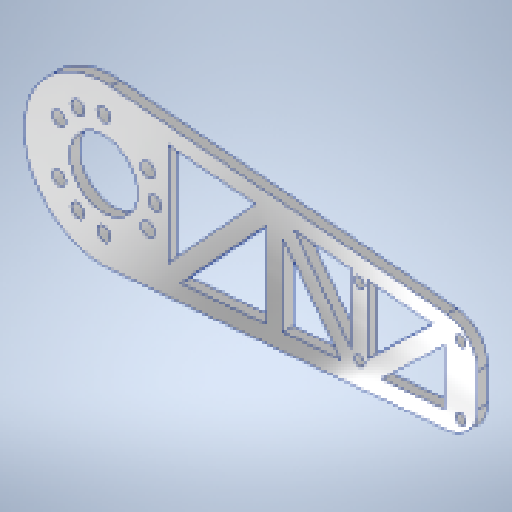
# Autodesk Inventor part: link1plate4
Saved by Autodesk Inventor 2024 (Build 280153000, 153)
## iProperties
Created: 2025-02-07
Part Number: link1plate4
Material: アルミニウム 6061
Document SubType Name: Modeling
Designer: tanoue_kota
Mass: 24.6432 g
Surface Area: 89.3933 cm^2
Volume: 9.1271 cm^3
Density: 2.7 g/cm^3
Appearance: アルミニウム - フラット
Author: tanoue_kota
Autodesk Inventor part; units mm, degrees
ref_plane "YZ Plane" through (0, 0, 0) normal (1, 0, 0) x (0, 1, 0)
ref_plane "XZ Plane" through (0, 0, 0) normal (0, 1, 0) x (-1, 0, 0)
ref_plane "XY Plane" through (0, 0, 0) normal (0, 0, 1) x (1, 0, 0)
sketch "スケッチ1" plane through (0, 0, 0) normal (0, 0, 1) x (1, 0, 0)
  line L0 (0, 0) -> (-57.5, 0)
  line L1 (-57.5, 0) -> (-57.5, 28)
  line L2 (-57.5, 28) -> (0, 28)
  line L3 (0, 28) -> (0, 0)
  line L4 (0, 14) -> (-110.5, 14)
  circle A0 centre (-110.5, 14) radius 53
  circle A1 centre (-110.5, 14) radius 23.5
  line L5 (0, 28) -> (-108.4685, 37.412)
  line L6 (0, 0) -> (-108.4685, -9.412)
  point P0 (-108.4685, -9.412)
  dimension "d3" = 47
  dimension "d0" = 28
  dimension "d1" = 57.5
  dimension "d2" = 106
  constraints: 14 end point, 2 coincident, 2 horizontal, 2 parallel, 1 centre point, 1 midpoint, 1 perpendicular, 1 symmetric about line, 1 tangent, 4 other
  measures "d0" distance of L2.end L0.start
  measures "d1" distance of L1.end L2.end
  measures "d2" diameter of A0
extrude "押し出し1" add sketch "スケッチ1" along normal blind 3 contours L6 A0 L1 L0 | L0 L1 L4 L3 | L4 L1 L2 L3 | L6 A1 L4 A0 | A0 L5 L2 L1 | L4 A1 L5 A0 | A1
sketch "スケッチ2" plane through (0, 0, 3) normal (0, 0, 1) x (1, 0, 0)
  line L0 (0, 28) -> (-108.4685, 37.412) projected
  line L1 (0, 28) -> (-47.5, 28)
  line L2 (-47.5, 28) -> (-47.5, 0)
  line L3 (-47.5, 0) -> (0, 0)
  line L4 (0, 0) -> (0, 28)
  line L5 (-5, 28) -> (-5, 0)
  line L6 (-35, 28) -> (-35, 0)
  line L7 (0, 14) -> (-47.5, 14)
  point P0 (-35, 24)
  point P1 (-5, 24)
  point P2 (-35, 4)
  point P3 (-5, 4)
  dimension "d6" = 28
  dimension "d7" = 47.5
  dimension "d8" = 5
  dimension "d9" = 30
  dimension "d10" = 10
  dimension "d11" = 10
  constraints: 14 end point, 6 point on line, 3 perpendicular, 2 midpoint, 2 parallel, 2 symmetric about line, 1 horizontal
  measures "d6" distance between parallel lines of L1 L3
  measures "d7" distance between parallel lines of L4 L2
  measures "d8" distance between parallel lines of L4 L5
  measures "d9" distance between parallel lines of L5 L6
  measures "d10" distance from line of L7 point (-5, 24)
  measures "d11" distance from line of L7 point (-35, 24)
hole "穴1" at (-35, 24, 3) at (-5, 24, 3) at (-35, 4, 3) at (-5, 4, 3) direction (0, 0, -1) diameter 3.1 end through all
sketch "スケッチ3" plane through (0, 0, 3) normal (0, 0, 1) x (1, 0, 0)
  arc A0 (-108.4685, 37.412) -> (-108.4685, -9.412) centre (-110.5, 14) ccw projected
  circle A1 centre (-110.5, 14) radius 15.18
  circle A2 centre (-110.5, 14) radius 6
  line L0 (-110.5, 14) -> (-118.09, 27.1463)
  line L1 (-123.6463, 21.59) -> (-110.5, 14)
  line L2 (-110.5, 14) -> (-102.91, 27.1463)
  line L3 (-110.5, 14) -> (-110.5, 29.18)
  point P0 (0, 0)
  point P1 (-123.6463, 6.41)
  point P2 (-110.5, -1.18)
  point P3 (-97.3537, 6.41)
  point P4 (-97.3537, 21.59)
  point P5 (-110.5, 29.18)
  point P6 (-118.09, 0.8537)
  point P7 (-95.32, 14)
  dimension "d19" = 30.36
  dimension "d22" = 360
  dimension "d24" = 12
  dimension "d28" = 360
  dimension "d59" = 30
  dimension "d61" = 30
  constraints: 8 end point, 4 coincident, 4 point on circle, 2 centre point, 1 perpendicular, 1 vertical, 11 other
  measures "d19" diameter of A1
  measures "d24" diameter of A2
  measures "d59" angle of L0 L1
  measures "d61" angle of L3 L2
hole "穴2" at (-123.6463, 21.59, 3) at (-123.6463, 6.41, 3) at (-110.5, -1.18, 3) at (-97.3537, 6.41, 3) at (-97.3537, 21.59, 3) at (-110.5, 29.18, 3) at (-118.09, 27.1463, 3) at (-118.09, 0.8537, 3) at (-95.32, 14, 3) direction (0, 0, -1) diameter 4.1 end through all
sketch "スケッチ4" plane through (0, 0, 3) normal (0, 0, 1) x (1, 0, 0)
  arc A0 (-108.4685, 37.412) -> (-108.4685, -9.412) centre (-110.5, 14) ccw projected
  circle A1 centre (-110.5, 14) radius 10
  circle A2 centre (-110.5, 14) radius 23.5
  line L0 (-94.4636, -3.178) -> (0, 5.0188)
  line L1 (0, 0) -> (0, 28) projected
  line L2 (-108.4685, -9.412) -> (0, 0) projected
  line L3 (-94.4636, 31.178) -> (0, 22.9812)
  line L4 (0, 28) -> (-108.4685, 37.412) projected
  line L5 (-10, 23.8489) -> (-10, 4.1511)
  line L6 (-37.5, 26.2352) -> (-37.5, 1.7648)
  circle A3 centre (-35, 4) radius 1.55 projected
  line L7 (-32.5, 25.8013) -> (-32.5, 2.1987)
  circle A4 centre (-35, 24) radius 1.55 projected
  line L8 (-10, 23.8489) -> (-32.5, 2.1987)
  line L9 (-32.5, 5.6681) -> (-13.3073, 24.1359)
  line L10 (-28.537, 2.5426) -> (-10, 20.3795)
  line L11 (-62.5, 28.4045) -> (-62.5, -0.4045)
  line L12 (-57.5, 27.9706) -> (-57.5, 0.0294)
  line L13 (-57.5, 27.9706) -> (-37.5, 1.7648)
  line L14 (-57.5, 23.8499) -> (-40.4496, 1.5089)
  line L15 (-54.1321, 27.6784) -> (-37.5, 5.8856)
  line L16 (-94.4636, 31.178) -> (-94.4636, -3.178)
  line L17 (-91.4636, 30.9177) -> (-91.4636, -2.9177)
  line L18 (-62.5, 28.4045) -> (-91.4636, -2.9177)
  line L19 (-91.4636, 0.7646) -> (-65.6521, 28.678)
  line L20 (-87.7615, -2.5965) -> (-62.5, 24.7222)
  dimension "d37" = 20
  dimension "d38" = 5
  dimension "d39" = 5
  dimension "d40" = 10
  dimension "d41" = 2.5
  dimension "d42" = 2.5
  dimension "d43" = 2.5
  dimension "d44" = 2.5
  dimension "d45" = 5
  dimension "d46" = 20
  dimension "d47" = 2.5
  dimension "d48" = 2.5
  dimension "d49" = 3
  dimension "d50" = 2.5
  dimension "d51" = 2.5
  constraints: 32 end point, 8 parallel, 8 point on line, 4 vertical, 3 point on circle, 2 centre point, 2 coincident, 26 other
  measures "d37" diameter of A1
  measures "d40" distance between parallel lines of L1 L5
  measures "d41" distance from line of A3.centre L6
  measures "d42" distance from line of A4.centre L7
  measures "d43" distance between parallel lines of L8 L9
  measures "d44" distance between parallel lines of L8 L10
  measures "d45" distance between parallel lines of L11 L12
  measures "d46" distance between parallel lines of L6 L12
  measures "d47" distance between parallel lines of L13 L14
  measures "d48" distance between parallel lines of L13 L15
  measures "d49" distance between parallel lines of L16 L17
  measures "d50" distance between parallel lines of L18 L19
  measures "d51" distance between parallel lines of L18 L20
extrude "押し出し2" cut sketch "スケッチ4" against normal blind 3 contours L17 L3 L19 A2 | A2 L19 L17 | L20 L11 L0 | L0 L10 L5 | L9 L7 L3 | L12 L14 L0 | L3 L6 L15 picked at (-90.6492, 17.3589)
fillet "フィレット1" radius 10 2 edges at (0, 28, 1.5) (0, 0, 1.5)
sketch "スケッチ5" plane through (0, 0, 3) normal (0, 0, 1) x (1, 0, 0)
  arc A0 (-108.4685, 37.412) -> (-108.4685, -9.412) centre (-110.5, 14) ccw projected
  circle A1 centre (-110.5, 14) radius 10
  point P0 (0, 0)
  dimension "d55" = 20
  constraints: 1 centre point, 1 coincident
  measures "d55" diameter of A1
extrude "押し出し3" cut sketch "スケッチ5" against normal blind 3
